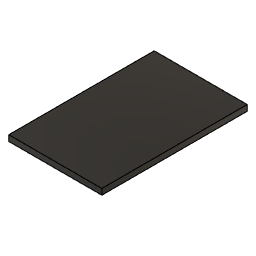
yeux v2 (Autodesk Fusion 360 design; units mm, degrees)
Autodesk Fusion 360 part; units mm, degrees
sketch "Esquisse1" plane through (0, 0, 0) normal (0, 0, 1) x (1, 0, 0)
  line L0 (8, 12.5) -> (-8, 12.5)
  line L1 (-8, 12.5) -> (-8, -12.5)
  line L2 (-8, -12.5) -> (8, -12.5)
  line L3 (8, -12.5) -> (8, 12.5)
  line L4 (8, 12.5) -> (-8, -12.5) construction
  line L5 (-8, 12.5) -> (8, -12.5) construction
  dimension "d1" = 16
  dimension "d2" = 25
  constraint horizontal L0
  constraint perpendicular L0 L1
  constraint parallel L0 L2
  constraint parallel L1 L3
  constraint coincident L4 origin
  constraint coincident L5 origin
  measures "d1" distance of L1.end L2.end
  measures "d2" distance of L0.end L1.end
sketch "Esquisse2" plane through (0, 0, 0) normal (0, 0, 1) x (1, 0, 0)
  line L0 (8, 12.5) -> (-8, 12.5)
  line L1 (-8, 12.5) -> (-8, -12.5)
  line L2 (-8, -12.5) -> (8, -12.5)
  line L3 (8, -12.5) -> (8, 12.5)
  line L4 (8, 12.5) -> (-8, -12.5) construction
  line L5 (-8, 12.5) -> (8, -12.5) construction
  dimension "d5" = 16
  dimension "d6" = 25
  constraint horizontal L0
  constraint perpendicular L0 L1
  constraint parallel L0 L2
  constraint parallel L1 L3
  constraint coincident L4 origin
  constraint coincident L5 origin
  measures "d5" distance of L1.end L2.end
  measures "d6" distance of L0.end L1.end
extrude "Extrusion2" add sketch "Esquisse2" along normal blind 1
sketch "Esquisse3" plane through (0, 0, 1) normal (0, 0, 1) x (-1, 0, 0)
  line L0 (-8, 12.5) -> (-8, -12.5)
  line L1 (-8, -12.5) -> (8, -12.5)
  line L2 (8, -12.5) -> (8, 12.5)
  line L3 (8, 12.5) -> (-8, 12.5)
  line L4 (-2.475, 3.475) -> (2.475, 3.475)
  line L5 (2.475, 3.475) -> (2.475, -3.475)
  line L6 (2.475, -3.475) -> (-2.475, -3.475)
  line L7 (-2.475, -3.475) -> (-2.475, 3.475)
  line L8 (-2.475, 3.475) -> (2.475, -3.475) construction
  line L9 (2.475, 3.475) -> (-2.475, -3.475) construction
  dimension "d9" = 4.95
  dimension "d10" = 6.95
  constraint horizontal L4
  constraint perpendicular L4 L5
  constraint parallel L4 L6
  constraint parallel L5 L7
  constraint coincident L8 origin
  constraint coincident L9 origin
  measures "d9" distance of L5.end L6.end
  measures "d10" distance of L4.end L5.end
extrude "Extrusion3" add sketch "Esquisse3" against normal blind 2.49 contours L4 L5 L6 L7
